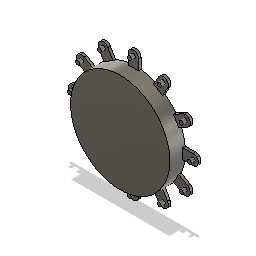
aft_spray_mask_75mm_flange (Autodesk Fusion 360 design; units mm, degrees)
Autodesk Fusion 360 part; units mm, degrees
sketch "Sketch1" plane through (0, 0, 0) normal (0, 0, 1) x (1, 0, 0)
  circle A0 centre (0, 0) radius 38.1
  circle A1 centre (0, 0) radius 46 construction
  circle A2 centre (0, 46) radius 4
  line L0 (-3.9962, 45.8261) -> (-3.9962, 37.8898)
  line L1 (3.9962, 45.8261) -> (3.9962, 37.8898)
  circle A3 centre (0, 46) radius 1.5
  line L2 (-19.4522, 41.6847) -> (-15.4841, 34.8117)
  line L3 (-26.3739, 37.6884) -> (-22.4057, 30.8155)
  circle A4 centre (-23, 39.8372) radius 4
  circle A5 centre (-23, 39.8372) radius 1.5
  line L4 (-37.6884, 26.3739) -> (-30.8155, 22.4057)
  line L5 (-41.6847, 19.4522) -> (-34.8117, 15.4841)
  circle A6 centre (-39.8372, 23) radius 4
  circle A7 centre (-39.8372, 23) radius 1.5
  line L6 (-45.8261, 3.9962) -> (-37.8898, 3.9962)
  line L7 (-45.8261, -3.9962) -> (-37.8898, -3.9962)
  circle A8 centre (-46, 0) radius 4
  circle A9 centre (-46, 0) radius 1.5
  line L8 (-41.6847, -19.4522) -> (-34.8117, -15.4841)
  line L9 (-37.6884, -26.3739) -> (-30.8155, -22.4057)
  circle A10 centre (-39.8372, -23) radius 4
  circle A11 centre (-39.8372, -23) radius 1.5
  line L10 (-26.3739, -37.6884) -> (-22.4057, -30.8155)
  line L11 (-19.4522, -41.6847) -> (-15.4841, -34.8117)
  circle A12 centre (-23, -39.8372) radius 4
  circle A13 centre (-23, -39.8372) radius 1.5
  line L12 (-3.9962, -45.8261) -> (-3.9962, -37.8898)
  line L13 (3.9962, -45.8261) -> (3.9962, -37.8898)
  circle A14 centre (0, -46) radius 4
  circle A15 centre (0, -46) radius 1.5
  line L14 (19.4522, -41.6847) -> (15.4841, -34.8117)
  line L15 (26.3739, -37.6884) -> (22.4057, -30.8155)
  circle A16 centre (23, -39.8372) radius 4
  circle A17 centre (23, -39.8372) radius 1.5
  line L16 (37.6884, -26.3739) -> (30.8155, -22.4057)
  line L17 (41.6847, -19.4522) -> (34.8117, -15.4841)
  circle A18 centre (39.8372, -23) radius 4
  circle A19 centre (39.8372, -23) radius 1.5
  line L18 (45.8261, -3.9962) -> (37.8898, -3.9962)
  line L19 (45.8261, 3.9962) -> (37.8898, 3.9962)
  circle A20 centre (46, 0) radius 4
  circle A21 centre (46, 0) radius 1.5
  line L20 (41.6847, 19.4522) -> (34.8117, 15.4841)
  line L21 (37.6884, 26.3739) -> (30.8155, 22.4057)
  circle A22 centre (39.8372, 23) radius 4
  circle A23 centre (39.8372, 23) radius 1.5
  line L22 (26.3739, 37.6884) -> (22.4057, 30.8155)
  line L23 (19.4522, 41.6847) -> (15.4841, 34.8117)
  circle A24 centre (23, 39.8372) radius 4
  circle A25 centre (23, 39.8372) radius 1.5
  dimension "d374" = 76.2
  dimension "d375" = 92
  dimension "d376" = 8
  dimension "d377" = 3
  dimension "d379" = 360
  constraint coincident A0.centre A1.centre
  constraint coincident A1 A2.centre
  constraint vertical A0.centre A2.centre
  constraint vertical L0
  constraint coincident A2 L0.start
  constraint coincident A1 L0.start
  constraint coincident A0 L0.end
  constraint vertical L1
  constraint coincident A2 L1.start
  constraint coincident A1 L1.start
  constraint coincident A0 L1.end
  constraint concentric A2 A3
  measures "d374" diameter of A0
  measures "d375" diameter of A1
  measures "d376" diameter of A2
  measures "d377" diameter of A3
extrude "Extrude1" add sketch "Sketch1" along normal blind 2 contours A0 | A0 L18 L19 A20 | A0 L20 L21 A22 | A20 | A0 L16 L17 A18 | A22 | A18 | A0 L22 L23 A24 | A0 L14 L15 A16 | A24 | A16 | A0 A2 L0 L1 | A0 L12 L13 A14 | A2 | A14 | A0 L2 L3 A4 | A0 L10 L11 A12 | A4 | A12 | A0 L4 L5 A6 | A0 L8 L9 A10 | A6 | A10 | A0 L6 L7 A8 | A8 | A3 | A5 | A7 | A9 | A11 | A13 | A15 | A17 | A19 | A21 | A23 | A25
extrude "Extrude2" add sketch "Sketch1" along normal blind 10 from surface at 2 contours A0
extrude "Extrude3" add sketch "Sketch1" along normal blind 3 from surface at 2 contours A3 | A5 | A7 | A9 | A11 | A13 | A15 | A17 | A19 | A21 | A23 | A25
equation "d374 = mmt_id"
equation "mmt_id = 76.2 mm" comment "LOC 75mm MMT"
